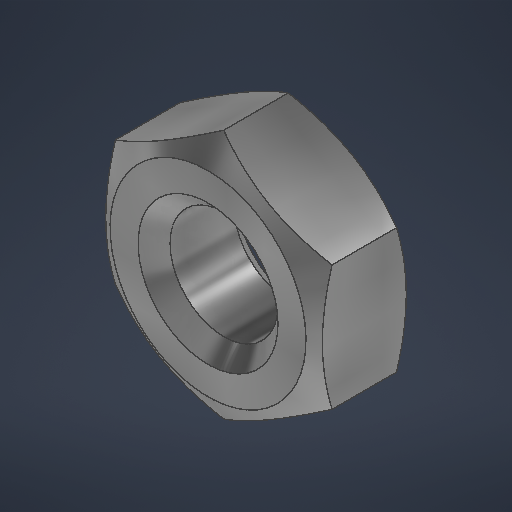
# Autodesk Inventor part: Гайка М3
Saved by Autodesk Inventor 2025 (Build 290162010, 162A)
## iProperties
Created: 2025-01-11
Part Number: Гайка М3
Material: Типовые
Document SubType Name: Modeling
Designer: Edward_Higgins
Density: 1 g/cm^3
Appearance: По умолчанию
Author: Edward_Higgins
Autodesk Inventor part; units mm, degrees
ref_plane "YZ Plane" through (0, 0, 0) normal (1, 0, 0) x (0, 1, 0)
ref_plane "XZ Plane" through (0, 0, 0) normal (0, 1, 0) x (-1, 0, 0)
ref_plane "XY Plane" through (0, 0, 0) normal (0, 0, 1) x (1, 0, 0)
sketch "Эскиз1" plane through (0, 0, 0) normal (0, 0, 1) x (1, 0, 0)
  circle A0 centre (0, 0) radius 1.35
  line L0 (0, 3.1292) -> (2.71, 1.5646)
  line L1 (2.71, 1.5646) -> (2.71, -1.5646)
  line L2 (2.71, -1.5646) -> (0, -3.1292)
  line L3 (0, -3.1292) -> (-2.71, -1.5646)
  line L4 (-2.71, -1.5646) -> (-2.71, 1.5646)
  line L5 (-2.71, 1.5646) -> (0, 3.1292)
  dimension "d0" = 2.7
  dimension "d1" = 5.42
  constraints: 12 end point, 2 coincident, 1 centre point, 1 vertical, 13 other
  measures "d0" diameter of A0
  measures "d1" distance between parallel lines of L1 L4
extrude "Выдавливание1" add sketch "Эскиз1" along normal mid plane 2.4
chamfer "Фаска1" distance 0.4 angle 45 2 edges at (-1.35, 0, 1.2) (-1.35, 0, -1.2)
sketch "Эскиз2" plane through (0, 0, 0) normal (1, 0, 0) x (0, 1, 0)
  line L0 (0, -4.7585) -> (0, 2.7781)
  line L1 (3.1292, -1.2) -> (3.1292, 1.2) projected
  line L2 (1.5646, 1.2) -> (3.1292, 1.2) projected
  line L3 (1.5646, -1.2) -> (1.5646, 1.2) projected
  line L4 (3.1292, -1.2) -> (1.5646, -1.2) projected
  line L5 (3.1292, 0.8083) -> (2.4508, 1.2)
  point P0 (0, 0)
  dimension "d7" = 30
  constraints: 4 end point, 3 point on line, 1 vertical
  measures "d7" angle of L2 L5
revolve "Вращение1" cut sketch "Эскиз2" angle 360 about axis through (0, 0, -4.7585) along (0, 0, 1) contours L5 L2 L1
mirror "Зеркальное отражение1" about plane through (0, 0, 0) normal (0, 0, 1) of "Вращение1"
